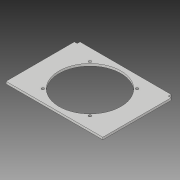
# Autodesk Inventor part: PowerSupplyEncEnds
Saved by Autodesk Inventor 2019 (Build 230136000, 136)
## iProperties
Created: 2021-08-16
Part Number: PowerSupplyEncEnds
Material: Generic
Document SubType Name: Modeling
Designer: devon
Density: 1 g/cm^3
Appearance: Default
Author: devon
Autodesk Inventor part; units mm, degrees
ref_plane "YZ Plane" through (0, 0, 0) normal (1, 0, 0) x (0, 1, 0)
ref_plane "XZ Plane" through (0, 0, 0) normal (0, 1, 0) x (-1, 0, 0)
ref_plane "XY Plane" through (0, 0, 0) normal (0, 0, 1) x (1, 0, 0)
sketch "Sketch1" plane through (0, 0, 0) normal (0, 1, 0) x (-1, 0, 0)
  line L0 (107.95, 79.375) -> (-107.95, 79.375)
  line L1 (-107.95, 79.375) -> (-107.95, -79.375)
  line L2 (-107.95, -79.375) -> (107.95, -79.375)
  line L3 (107.95, -79.375) -> (107.95, 79.375)
  line L4 (107.95, 79.375) -> (-107.95, -79.375) construction
  line L5 (-107.95, 79.375) -> (107.95, -79.375) construction
  point P0 (0, 0)
  dimension "d0" = 215.9
  dimension "d1" = 158.75
  constraints: 12 end point, 2 midpoint, 2 parallel, 1 horizontal, 1 perpendicular
  measures "d0" distance of L1.end L2.end
  measures "d1" distance of L2.end L0.start
extrude "Extrusion1" add sketch "Sketch1" along normal blind 5
sketch "Sketch2" plane through (0, 5, 0) normal (0, 1, 0) x (1, 0, 0)
  line L0 (107.95, 79.375) -> (-107.95, 79.375) projected
  line L1 (-107.95, 79.375) -> (-101.6, 79.375)
  line L2 (-101.6, 79.375) -> (-101.6, 73.025)
  line L3 (-101.6, 73.025) -> (-107.95, 73.025)
  line L4 (-107.95, 73.025) -> (-107.95, 79.375)
  line L5 (107.95, 79.375) -> (101.6, 79.375)
  line L6 (101.6, 79.375) -> (101.6, 73.025)
  line L7 (101.6, 73.025) -> (107.95, 73.025)
  line L8 (107.95, 73.025) -> (107.95, 79.375)
  point P0 (0, 0)
  dimension "d4" = 6.35
  dimension "d5" = 6.35
  dimension "d6" = 6.35
  dimension "d7" = 6.35
  constraints: 16 end point, 4 parallel, 2 horizontal, 2 perpendicular
  measures "d4" distance of L1.end L2.end
  measures "d5" distance of L2.end L3.end
  measures "d6" distance of L5.end L6.end
  measures "d7" distance of L6.end L7.end
extrude "Extrusion2" cut sketch "Sketch2" against normal up to next
sketch "Sketch3" plane through (0, 5, 0) normal (0, 1, 0) x (1, 0, 0)
  point P0 (0, 0)
  point P1 (-52.5, 52.5)
  point P2 (-52.5, -52.5)
  point P3 (52.5, -52.5)
  point P4 (52.5, 52.5)
  dimension "d17" = 105
  dimension "d18" = 105
  dimension "d19" = 52.5
  dimension "d20" = 52.5
  dimension "d21" = 105
  dimension "d22" = 52.5
  dimension "d23" = 105
  dimension "d24" = 52.5
  measures "d17" distance of point (52.5, 52.5) point (-52.5, 52.5)
  measures "d18" distance of point (-52.5, -52.5) point (-52.5, 52.5)
  measures "d19" horizontal distance of point (0, 0) point (-52.5, -52.5)
  measures "d20" horizontal distance of point (0, 0) point (-52.5, 52.5)
  measures "d21" distance of point (-52.5, -52.5) point (52.5, -52.5)
  measures "d22" horizontal distance of point (0, 0) point (52.5, 52.5)
  measures "d23" distance of point (52.5, 52.5) point (52.5, -52.5)
  measures "d24" horizontal distance of point (0, 0) point (-52.5, 52.5)
hole "Hole1" at (-52.5, 5, -52.5) at (-52.5, 5, 52.5) at (52.5, 5, 52.5) at (52.5, 5, -52.5) direction (0, -1, 0) diameter 6 depth 10.9728 tip angle 118
sketch "Sketch4" plane through (0, 5, 0) normal (0, 1, 0) x (1, 0, 0)
  circle A0 centre (0, 0) radius 69
  dimension "d25" = 138
  constraints: 1 centre point, 1 coincident
  measures "d25" diameter of A0
extrude "Extrusion3" cut sketch "Sketch4" against normal up to next
body "Solid1"
